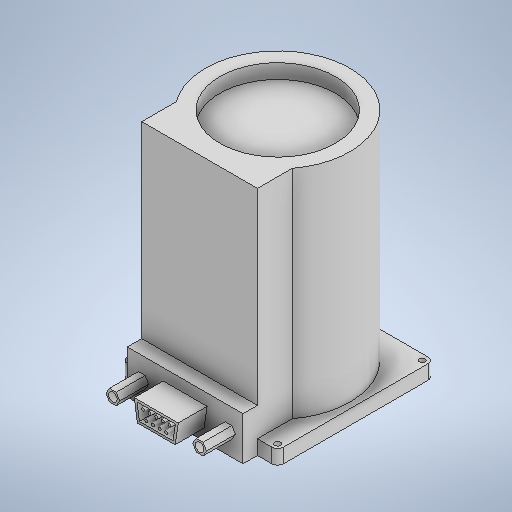
# Autodesk Inventor part: sensor 1
Saved by Autodesk Inventor 2025 (Build 290162000, 162)
## iProperties
Created: 2024-04-10
Part Number: sensor 1
Material: Generic
Document SubType Name: Modeling
Designer: mahal
Density: 1 g/cm^3
Appearance: Default
Author: mahal
Autodesk Inventor part; units mm, degrees
sketch "Sketch1" plane through (0, 0, 0) normal (0, 1, 0) x (-1, 0, 0)
  line L0 (27, 27) -> (-27, 27)
  line L1 (-27, 27) -> (-27, -27)
  line L2 (-27, -27) -> (27, -27)
  line L3 (27, -27) -> (27, 27)
  line L4 (27, 27) -> (-27, -27) construction
  line L5 (-27, 27) -> (27, -27) construction
  circle A0 centre (25, 25) radius 1
  circle A1 centre (25, -25) radius 1
  circle A2 centre (-25, -25) radius 1
  circle A3 centre (-25, 25) radius 1
  point P0 (0, 0)
  dimension "d0" = 54
  dimension "d1" = 54
  dimension "d2" = 2
  dimension "d3" = 2
  dimension "d4" = 2
  dimension "d5" = 2
  constraints: 12 end point, 4 centre point, 3 point on line, 2 midpoint, 2 parallel, 1 horizontal, 1 perpendicular
  measures "d0" distance of L2.end L1.end
  measures "d1" distance of L1.end L0.end
  measures "d2" diameter of A0
  measures "d3" diameter of A1
  measures "d4" diameter of A2
  measures "d5" diameter of A3
extrude "Extrusion1" add sketch "Sketch1" along normal blind 5
fillet "Fillet1" radius 2 1 edges at (27, 2.5, -27)
fillet "Fillet2" radius 2 3 edges at (-27, 2.5, -27) (-27, 2.5, 27) (27, 2.5, 27)
ref_plane "Work Plane1" through (0, 5, 0) normal (0, 1, 0) x (1, 0, 0)
sketch "Sketch3" plane through (0, 5, 0) normal (0, 1, 0) x (1, 0, 0)
  circle A0 centre (0, 0) radius 25
  line L0 (-25, -27) -> (25, -27) projected
  line L1 (0, -27) -> (20, -27)
  line L2 (20, -27) -> (20, -15)
  line L3 (0, -27) -> (-20, -27)
  line L4 (-20, -27) -> (-20, -15)
  dimension "d11" = 50
  dimension "d12" = 20
  dimension "d13" = 20
  constraints: 8 end point, 2 perpendicular, 2 point on circle, 2 point on line, 1 centre point, 1 coincident, 1 midpoint
  measures "d11" diameter of A0
  measures "d12" distance of L1.start L1.end
  measures "d13" distance of L1.start L3.end
extrude "Extrusion2" add sketch "Sketch3" along normal blind 75
ref_plane "Work Plane2" through (0, 80, 0) normal (0, 1, 0) x (1, 0, 0)
sketch "Sketch4" plane through (0, 80, 0) normal (0, 1, 0) x (1, 0, 0)
  circle A0 centre (0, 0) radius 20
  dimension "d17" = 40
  constraints: 1 centre point, 1 coincident
  measures "d17" diameter of A0
extrude "Extrusion3" cut sketch "Sketch4" against normal blind 5
ref_plane "Work Plane3" through (-25, 0, 27) normal (0, 0, 1) x (1, 0, 0)
sketch "Sketch5" plane through (-25, 0, 27) normal (0, 0, 1) x (1, 0, 0)
  line L0 (25, 0) -> (25, 7.5)
  line L1 (5, 15) -> (45, 15)
  line L2 (45, 15) -> (45, 0)
  line L3 (45, 0) -> (5, 0)
  line L4 (5, 0) -> (5, 15)
  line L5 (5, 15) -> (45, 0) construction
  line L6 (45, 15) -> (5, 0) construction
  dimension "d21" = 7.5
  dimension "d22" = 40
  dimension "d23" = 15
  constraints: 14 end point, 2 midpoint, 2 parallel, 1 horizontal, 1 perpendicular, 1 vertical
  measures "d21" distance of L0.start L0.end
  measures "d22" distance of L2.end L3.end
  measures "d23" distance of L1.end L2.end
extrude "Extrusion4" add sketch "Sketch5" along normal blind 5
ref_plane "Work Plane4" through (-25, 0, 32) normal (0, 0, 1) x (1, 0, 0)
sketch "Sketch6" plane through (-25, 0, 32) normal (0, 0, 1) x (1, 0, 0)
  line L0 (25, 7.5) -> (25, 8.92)
  circle A0 centre (25, 8.92) radius 0.5
  line L1 (25, 8.92) -> (27.3, 8.92)
  line L2 (27.3, 8.92) -> (29.6, 8.92)
  line L3 (25, 8.92) -> (22.7, 8.92)
  line L4 (22.7, 8.92) -> (20.4, 8.92)
  circle A1 centre (20.4, 8.92) radius 0.5
  circle A2 centre (27.3, 8.92) radius 0.5
  circle A3 centre (22.7, 8.92) radius 0.5
  circle A4 centre (29.6, 8.92) radius 0.5
  line L5 (25, 7.5) -> (25, 6.08)
  line L6 (26.15, 6.08) -> (25, 6.08)
  line L7 (23.85, 6.08) -> (25, 6.08)
  circle A5 centre (26.15, 6.08) radius 0.5
  circle A6 centre (23.85, 6.08) radius 0.5
  line L8 (23.85, 6.08) -> (21.55, 6.08)
  line L9 (26.15, 6.08) -> (28.45, 6.08)
  circle A7 centre (28.45, 6.08) radius 0.5
  circle A8 centre (21.55, 6.08) radius 0.5
  line L10 (18.3522, 10.2186) -> (31.6478, 10.2186)
  line L11 (30.8187, 4.7814) -> (19.1813, 4.7814)
  line L12 (31.6478, 10.2186) -> (30.8187, 4.7814)
  line L13 (18.3522, 10.2186) -> (19.1813, 4.7814)
  line L14 (25, 10.2186) -> (25, 11.0186)
  line L15 (25, 4.7814) -> (25, 3.9814)
  line L16 (25, 3.9814) -> (31.5285, 3.9814)
  line L17 (31.5285, 3.9814) -> (32.5973, 11.0186)
  line L18 (32.5973, 11.0186) -> (25, 11.0186)
  line L19 (25, 3.9814) -> (18.4715, 3.9814)
  line L20 (18.4715, 3.9814) -> (17.4027, 11.0186)
  line L21 (17.4027, 11.0186) -> (25, 11.0186)
  point P0 (25, 0)
  dimension "d30" = 1
  dimension "d33" = 1
  dimension "d34" = 1
  dimension "d35" = 1
  dimension "d36" = 1
  dimension "d38" = 1
  dimension "d39" = 1
  dimension "d40" = 1
  dimension "d41" = 1
  dimension "d44" = 0.8
  constraints: 44 end point, 9 centre point, 9 coincident, 5 horizontal, 5 symmetric about line, 2 midpoint, 2 point on line, 2 vertical, 1 collinear, 1 parallel, 1 perpendicular
  measures "d30" diameter of A0
  measures "d33" diameter of A1
  measures "d34" diameter of A2
  measures "d35" diameter of A3
  measures "d36" diameter of A4
  measures "d38" diameter of A5
  measures "d39" diameter of A6
  measures "d40" diameter of A7
  measures "d41" diameter of A8
  measures "d44" distance of L15.start L15.end
extrude "Extrusion5" add sketch "Sketch6" along normal blind 10 contours A1 | A3 L4 L3 | L3 L4 A3 | A4 | A2 L2 L1 | L1 L2 A2 | A0 L3 L0 | L0 L1 A0 | A7 | A5 L9 L6 | L6 L9 A5 | A8 | A6 L8 L7 | L7 L8 A6 | L3 A0 L1 | L13 L11 L15 L19 L20 L21 L14 L10 | L14 L18 L17 L16 L15 L11 L12 L10
sketch "Sketch7" plane through (-25, 0, 32) normal (0, 0, 1) x (1, 0, 0)
  line L0 (5, 15) -> (5, 0) projected
  line L1 (5, 7.5) -> (10, 7.5)
  circle A0 centre (10, 7.5) radius 1.5
  line L2 (12.3579, 7.5) -> (11.1789, 5.458)
  line L3 (11.1789, 5.458) -> (8.8211, 5.458)
  line L4 (8.8211, 5.458) -> (7.6421, 7.5)
  line L5 (7.6421, 7.5) -> (8.8211, 9.542)
  line L6 (8.8211, 9.542) -> (11.1789, 9.542)
  line L7 (11.1789, 9.542) -> (12.3579, 7.5)
  line L8 (25, 0) -> (25, 2.1902)
  circle A1 centre (40, 7.5) radius 1.5
  line L9 (37.6421, 7.5) -> (38.8211, 5.458)
  line L10 (38.8211, 5.458) -> (41.1789, 5.458)
  line L11 (41.1789, 5.458) -> (42.3579, 7.5)
  line L12 (42.3579, 7.5) -> (41.1789, 9.542)
  line L13 (41.1789, 9.542) -> (38.8211, 9.542)
  line L14 (38.8211, 9.542) -> (37.6421, 7.5)
  dimension "d48" = 5
  dimension "d49" = 3
  constraints: 28 end point, 7 symmetric about line, 2 centre point, 2 coincident, 1 horizontal, 1 midpoint, 1 point on line, 1 vertical, 14 other
  measures "d48" distance of L1.start L1.end
  measures "d49" diameter of A0
extrude "Extrusion6" add sketch "Sketch7" along normal blind 10
body "Solid1"
